ad50acd6-c076-44dd-81ce-8105228f990e (Autodesk Fusion 360 design; units mm, degrees)
Autodesk Fusion 360 part; units mm, degrees
note: some values were not read from the file. Set by a fixed rule: which sketch regions a step uses.
sketch "Sketch1" plane through (0, 0, 0) normal (0, 1, 0) x (1, 0, 0)
  circle A0 centre (0, 0) radius 12.7
  circle A1 centre (0, 0) radius 14.351
  circle A2 centre (0, 0) radius 11.1125
  circle A3 centre (0, 0) radius 11.9341
  arc A4 (14.3142, -1.0267) -> (-13.1538, -5.7384) centre (0, 0) ccw
  circle A5 centre (0, 0) radius 1.9844
  line L0 (0, 0) -> (14.351, 0) construction
  line L1 (0, 0) -> (-1.0401, -11.8887)
  line L2 (0, 0) -> (-2.0723, -11.7528)
  line L3 (0, 0) -> (-3.0888, -11.5275)
  line L4 (0, 0) -> (-4.0817, -11.2144)
  line L5 (0, 0) -> (-5.0436, -10.816)
  line L6 (0, 0) -> (-5.967, -10.3352)
  line L7 (0, 0) -> (-6.8451, -9.7758)
  line L8 (-1.0401, -11.8887) -> (-0.0026, -11.9795) construction
  line L9 (-2.0723, -11.7528) -> (-0.0211, -12.1145) construction
  line L10 (-3.0888, -11.5275) -> (-0.0709, -12.3361) construction
  line L11 (-4.0817, -11.2144) -> (-0.1671, -12.6392) construction
  line L12 (-5.0436, -10.816) -> (-0.3242, -13.0166) construction
  line L13 (-5.967, -10.3352) -> (-0.5555, -13.4596) construction
  line L14 (-6.8451, -9.7758) -> (-0.8734, -13.9573) construction
  line L15 (0, 0) -> (-7.6711, -9.142)
  line L16 (-7.6711, -9.142) -> (-1.2887, -14.4975) construction
  line L17 (0, 0) -> (-8.4387, -8.4387)
  line L18 (-8.4387, -8.4387) -> (-1.811, -15.0664) construction
  spline S0 degree 5 poles (-1.811, -15.0664) (-1.7951, -15.0466) (-1.7631, -15.0074) (-1.7144, -14.9499) (-1.6482, -14.8758) (-1.5641, -14.7865) (-1.4798, -14.6995) (-1.3965, -14.6137) (-1.3155, -14.5278) (-1.2375, -14.4411) (-1.1631, -14.3531) (-1.0922, -14.264) (-1.0247, -14.174) (-0.96, -14.0836) (-0.8977, -13.9935) (-0.8373, -13.9041) (-0.7787, -13.8158) (-0.7217, -13.7286) (-0.6666, -13.6425) (-0.6136, -13.5573) (-0.5628, -13.4728) (-0.5145, -13.3891) (-0.4686, -13.3061) (-0.4253, -13.2239) (-0.3843, -13.1427) (-0.3455, -13.0628) (-0.309, -12.9843) (-0.2746, -12.9074) (-0.2423, -12.8321) (-0.2122, -12.7585) (-0.1843, -12.6866) (-0.1586, -12.6164) (-0.1352, -12.5483) (-0.1138, -12.4825) (-0.0944, -12.4192) (-0.0769, -12.3588) (-0.0613, -12.3013) (-0.0475, -12.2469) (-0.0358, -12.1954) (-0.0262, -12.1469) (-0.0188, -12.1014) (-0.0131, -12.0599) (-0.0086, -12.0234) (-0.0047, -11.9929) (-0.0012, -11.9694) (0.0016, -11.9524) (0.0024, -11.9431) (0.0017, -11.938) (0.0007, -11.9353) (0, -11.9341) knots 0 0 0 0 0 0 0.022222 0.044444 0.066667 0.088889 0.111111 0.133333 0.155556 0.177778 0.2 0.222222 0.244444 0.266667 0.288889 0.311111 0.333333 0.355556 0.377778 0.4 0.422222 0.444444 0.466667 0.488889 0.511111 0.533333 0.555556 0.577778 0.6 0.622222 0.644444 0.666667 0.688889 0.711111 0.733333 0.755556 0.777778 0.8 0.822222 0.844444 0.866667 0.888889 0.911111 0.933333 0.955556 0.977778 1 1 1 1 1 1
  line L19 (-1.908, -15.1875) -> (-1.7139, -14.9454)
  line L20 (0.0349, -11.9945) -> (-0.0349, -11.8736)
  line L21 (-0.1892, -12.6986) -> (0, 0)
  line L22 (0, 0) -> (-0.697, -6.1381) construction
  line L23 (0, -11.9341) -> (0, 0) construction
  spline S1 degree 5 poles (0, -11.9341) (0, -11.8779) (0, -11.776) (0, -11.654) (0, -11.5419) (0, -11.4371) (0, -11.3403) (0, -11.2401) (0, -11.1576) (0, -11.1125) knots 0 0 0 0 0 0 0.2 0.4 0.6 0.8 1 1 1 1 1 1
  spline S2 degree 5 poles (-2.6759, -11.6302) (-2.6633, -11.5755) (-2.6405, -11.4761) (-2.6131, -11.3572) (-2.588, -11.248) (-2.5645, -11.1459) (-2.5428, -11.0516) (-2.5203, -10.9539) (-2.5018, -10.8735) (-2.4917, -10.8295) knots 0 0 0 0 0 0 0.2 0.4 0.6 0.8 1 1 1 1 1 1
  line L24 (0, -12.0224) -> (0, -11.8458)
  line L25 (0, -11.1835) -> (0, -11.0415)
  line L26 (-2.6957, -11.7163) -> (-2.6561, -11.5442)
  line L27 (-2.5076, -10.8987) -> (-2.4758, -10.7604)
  spline S3 degree 5 poles (-1.6134, -15.0888) (-1.6245, -15.066) (-1.6469, -15.0206) (-1.6814, -14.9537) (-1.7293, -14.8666) (-1.7913, -14.7607) (-1.8539, -14.6571) (-1.9158, -14.5547) (-1.9755, -14.4529) (-2.0321, -14.3509) (-2.0849, -14.2485) (-2.1339, -14.1457) (-2.1796, -14.0428) (-2.2223, -13.9403) (-2.2629, -13.8385) (-2.3017, -13.7379) (-2.339, -13.6386) (-2.3749, -13.5409) (-2.4093, -13.4446) (-2.4419, -13.3496) (-2.4725, -13.256) (-2.5008, -13.1635) (-2.5269, -13.0723) (-2.5507, -12.9825) (-2.5725, -12.8943) (-2.5923, -12.8077) (-2.6103, -12.723) (-2.6266, -12.6403) (-2.6412, -12.5597) (-2.654, -12.4812) (-2.6651, -12.4048) (-2.6743, -12.3308) (-2.6819, -12.2591) (-2.688, -12.1902) (-2.6927, -12.1242) (-2.6962, -12.0613) (-2.6986, -12.0019) (-2.6998, -11.9457) (-2.6996, -11.8929) (-2.6981, -11.8434) (-2.6952, -11.7975) (-2.6914, -11.7557) (-2.6876, -11.7191) (-2.6845, -11.6886) (-2.6827, -11.6649) (-2.6816, -11.6477) (-2.6803, -11.6385) (-2.6785, -11.6336) (-2.6769, -11.6312) (-2.6759, -11.6302) knots 0 0 0 0 0 0 0.022222 0.044444 0.066667 0.088889 0.111111 0.133333 0.155556 0.177778 0.2 0.222222 0.244444 0.266667 0.288889 0.311111 0.333333 0.355556 0.377778 0.4 0.422222 0.444444 0.466667 0.488889 0.511111 0.533333 0.555556 0.577778 0.6 0.622222 0.644444 0.666667 0.688889 0.711111 0.733333 0.755556 0.777778 0.8 0.822222 0.844444 0.866667 0.888889 0.911111 0.933333 0.955556 0.977778 1 1 1 1 1 1
  line L28 (-1.546, -15.2286) -> (-1.6808, -14.9491)
  line L29 (-2.7235, -11.6813) -> (-2.6284, -11.5791)
  point P0 (-0.1892, -12.6986)
  point P1 (0, -11.1125)
  point P2 (-1.9948, -14.4173)
  point P3 (-2.2784, -13.7977)
  point P4 (-2.4766, -13.2414)
  point P5 (-2.6027, -12.7579)
  point P6 (-2.6711, -12.3548)
  point P7 (-2.697, -12.0379)
  point P8 (-2.6958, -11.8107)
  point P9 (-2.6835, -11.675)
  point P10 (-2.4917, -10.8295)
  dimension "d2" = 28.702
  dimension "id" = 22.225
  dimension "BaseDiameter" = 23.8682
  dimension "d1" = 3.9688
  dimension "d34" = 5
  dimension "d35" = 5
  dimension "d36" = 5
  dimension "d37" = 5
  dimension "d38" = 5
  dimension "d39" = 5
  dimension "d41" = 1.0414
  dimension "d42" = 2.0829
  dimension "d43" = 3.1243
  dimension "d44" = 4.1658
  dimension "d45" = 5.2072
  dimension "d46" = 6.2487
  dimension "d47" = 7.2901
  dimension "d48" = 5
  dimension "d49" = 8.3316
  dimension "d50" = 5
  dimension "d51" = 9.373
  dimension "d55" = 5.625
  dimension "d60" = 5
  constraint coincident A0.centre A1.centre
  constraint concentric A0 A2
  constraint coincident A1 A4.end
  constraint horizontal L0
  constraint coincident A4 L0.end
  constraint coincident A3 S0.end
  constraint coincident A3 L1.end
  constraint coincident A3 L2.end
  constraint coincident A3 L3.end
  constraint coincident A3 L4.end
  constraint coincident A3 L5.end
  constraint coincident A3 L6.end
  constraint coincident A3 L7.end
  constraint vertical A0.centre S0.end
  constraint tangent A3 L8
  constraint tangent A3 L9
  constraint tangent A3 L10
  constraint tangent A3 L11
  constraint tangent A3 L12
  constraint tangent A3 L13
  constraint tangent A3 L14
  constraint coincident A3 L15.end
  constraint tangent A3 L16
  constraint coincident A3 L17.end
  constraint tangent A3 L18
  constraint midpoint L18.end L19
  constraint midpoint S0.end L20
  constraint coincident A0 P0
  constraint coincident S0 P0
  constraint coincident P0 L21.start
  constraint coincident L23 P1
  constraint coincident A2 P1
  constraint coincident P1 S1.end
  constraint midpoint S0.end L24
  constraint midpoint P1 L25
  constraint symmetric S0.end L22 S2.start
  constraint symmetric L8.end L22 P9
  constraint symmetric L9.end L22 P8
  constraint symmetric L10.end L22 P7
  constraint symmetric L11.end L22 P6
  constraint symmetric L12.end L22 P5
  constraint symmetric L13.end L22 P4
  constraint symmetric L14.end L22 P3
  constraint symmetric L16.end L22 P2
  constraint symmetric L18.end L22 S3.start
  constraint symmetric L19.start L22 L28.start
  constraint symmetric L19.end L22 L28.end
  constraint symmetric L20.start L22 L29.start
  constraint symmetric L20.end L22 L29.end
  constraint symmetric L22 P1 P10
  constraint symmetric L22 L24.start L26.start
  constraint symmetric L22 L24.end L26.end
  constraint symmetric L22 L25.start L27.start
  constraint symmetric L22 L25.end L27.end
  constraint vertical L24
  constraint vertical L25
  measures "d2" diameter of A1
  measures "id" diameter of A2
  measures "BaseDiameter" diameter of A3
  measures "d1" diameter of A5
  measures "d34" angle of L1 L2
  measures "d35" angle of L2 L3
  measures "d36" angle of L3 L4
  measures "d37" angle of L4 L5
  measures "d38" angle of L5 L6
  measures "d39" angle of L6 L7
  measures "d41" distance of L1.end L8.end
  measures "d42" distance of L2.end L9.end
  measures "d43" distance of L3.end L10.end
  measures "d44" distance of L4.end L11.end
  measures "d45" distance of L5.end L12.end
  measures "d46" distance of L6.end L13.end
  measures "d47" distance of L7.end L14.end
  measures "d48" angle of L7 L15
  measures "d49" distance of L15.end L16.end
  measures "d50" angle of L15 L17
  measures "d51" distance of L17.end L18.end
  measures "d55" angle of L21 L22
  measures "d60" angle of L1 L23
extrude "Extrude1" add sketch "Sketch1" along normal blind 304.8 contours A0 A1 S0 S3 | A3 S0 L21 | A0 A3 L21 S3 | A2 A3 L21 S1 L24 L25 | A2 A3 L1 L21 | A2 A3 L2 S2 L26 L27 | A2 A3 L1 L2 makes body 1
pattern_circular "C-Pattern2" count 12 over 360 about axis through (0, 1.75, 0) along (0, 1, 0) of bodies 1 makes body 2 at (3.5228, 203.2, 10.5393) makes body 3 at (8.3205, 203.2, 7.3659) makes body 4 at (10.8887, 203.2, 2.2188) makes body 5 at (10.5393, 101.6, -3.5228) makes body 6 at (7.3659, 203.2, -8.3205) makes body 7 at (2.2188, 203.2, -10.8887) makes body 8 at (-3.5228, 203.2, -10.5393) makes body 9 at (-8.3205, 203.2, -7.3659) makes body 10 at (-10.8887, 203.2, -2.2188) makes body 11 at (-10.5393, 203.2, 3.5228) makes body 12 at (-7.3659, 203.2, 8.3205)
extrude "Extrude2" add sketch "Sketch1" along normal blind 304.8 contours A2 A5 L17 L21 | A2 A5 L1 L21 | A2 A5 L1 L2 | A2 A5 L2 L3 | A2 A5 L3 L4 | A2 A5 L15 L17 | A2 A5 L4 L5 | A2 A5 L7 L15 | A2 A5 L5 L6 | A2 A5 L6 L7 bodies 1 2 3 4 5 6 7 8 9 10 11 12
ref_plane "WorkPlane1" through (6.2747, 152.4, -0.8261) normal (0.130526, 0, 0.991445) x (0.991445, 0, -0.130526)
fillet "Fillet1" [suppressed]
mirror "Mirror3" [suppressed]
pattern_circular "C-Pattern1" [suppressed]
equation "d = 1 in"
equation "OutsideDiameter = d2"
equation "PitchDiameter = d"
equation "id = PitchDiameter - 2 * ( PitchDiameter / TeethNumber )"
equation "BaseDiameter = PitchDiameter * cos(20 deg)"
equation "Length = 12 in"
equation "t = 16"
equation "ShaftDiameter = d1"
equation "TeethNumber = t"
equation "Pitch = 32"
equation "d30 = ( 1.25 * ( PitchDiameter / TeethNumber ) ) - ( PitchDiameter / TeethNumber )"
equation "Basecircum = PI * PitchDiameter * cos(20 deg)"
equation "d41 = Basecircum * 5 / 360"
equation "d42 = Basecircum * 10 / 360"
equation "d43 = Basecircum * 15 / 360"
equation "d44 = Basecircum * 20 / 360"
equation "d45 = Basecircum * 25 / 360"
equation "d46 = Basecircum * 30 / 360"
equation "d47 = Basecircum * 35 / 360"
equation "d49 = Basecircum * 40 / 360"
equation "d51 = Basecircum * 45 / 360"
equation "d55 = ( 360 / ( 4 * TeethNumber ) ) * 1 deg"
